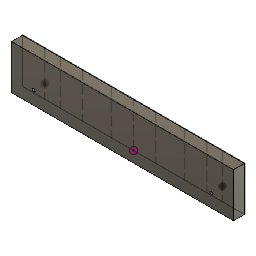
03part (Autodesk Fusion 360 design; units mm, degrees)
Autodesk Fusion 360 part; units mm, degrees
sketch "Sketch2" plane through (0, 0, 0) normal (0, 0, 1) x (1, 0, 0)
  line L0 (-250, 100) -> (250, 100)
  line L1 (250, 100) -> (250, 0)
  line L2 (250, 0) -> (-250, 0)
  line L3 (-250, 0) -> (-250, 100)
  line L4 (0, 0) -> (0, 100) construction
  line L5 (50, 100) -> (50, 0) construction
  line L6 (-50, 100) -> (-50, 0) construction
  line L7 (115, 100) -> (115, 0) construction
  line L8 (165, 100) -> (165, 0) construction
  line L9 (-115, 100) -> (-115, 0) construction
  line L10 (-165, 100) -> (-165, 0) construction
  line L11 (200, 100) -> (200, 0) construction
  line L12 (-200, 100) -> (-200, 0) construction
  circle A0 centre (200, 30) radius 3
  circle A1 centre (-200, 30) radius 3
  dimension "d6" = 500
  dimension "d7" = 100
  dimension "d8" = 100
  dimension "d9" = 50
  dimension "d10" = 330
  dimension "d11" = 200
  dimension "d12" = 6
  dimension "d13" = 30
  constraint horizontal L0
  constraint vertical L1
  constraint horizontal L2
  constraint vertical L3
  constraint midpoint L2 L4.start
  constraint coincident L4.start origin
  constraint midpoint L0 L4.end
  constraint coincident L0 L5.start
  constraint coincident L2 L5.end
  constraint perpendicular L2 L5
  constraint coincident L0 L6.start
  constraint coincident L2 L6.end
  constraint perpendicular L2 L6
  constraint coincident L0 L7.start
  constraint coincident L2 L7.end
  constraint perpendicular L2 L7
  constraint coincident L0 L8.start
  constraint coincident L2 L8.end
  constraint perpendicular L2 L8
  constraint coincident L0 L9.start
  constraint coincident L2 L9.end
  constraint perpendicular L2 L9
  constraint coincident L0 L10.start
  constraint coincident L2 L10.end
  constraint perpendicular L2 L10
  constraint coincident L0 L11.start
  constraint coincident L2 L11.end
  constraint perpendicular L2 L11
  constraint coincident L0 L12.start
  constraint coincident L2 L12.end
  constraint perpendicular L2 L12
  constraint symmetric L4 L11 L12
  constraint coincident L11 A0.centre
  constraint symmetric L4 A0 A1
  measures "d6" distance of L1.end L2.end
  measures "d7" distance of L0.start L2.end
  measures "d8" distance of L5 L6
  measures "d9" distance of L9 L10
  measures "d10" distance of L8 L10
  measures "d11" distance of L4 L11
  measures "d12" diameter of A0
  measures "d13" distance of L2 A0.centre
extrude "Extrude1" add sketch "Sketch2" along normal blind 25
